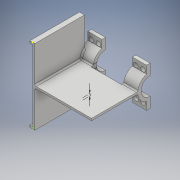
# Autodesk Inventor part: scopeHolderv2
Saved by Autodesk Inventor 2018 (Build 220112000, 112)
## iProperties
Created: 2019-03-22
Part Number: scopeHolderv2
Material: Generic
Document SubType Name: Modeling
Designer: Aditya Kendre
Density: 1 g/cm^3
Appearance: Default
Author: Aditya Kendre
## iProperties of the stored document scopeHolderv2_3DPrint.ipt
Created: 2019-03-22
Part Number: scopeHolderv2_3DPrint
Material: Generic
Document SubType Name: Modeling
Designer: Aditya Kendre
Density: 1 g/cm^3
Appearance: Default
Author: Aditya Kendre
Autodesk Inventor part; units mm, degrees
ref_plane "YZ Plane" through (0, 0, 0) normal (1, 0, 0) x (0, 1, 0)
ref_plane "XZ Plane" through (0, 0, 0) normal (0, 1, 0) x (-1, 0, 0)
ref_plane "XY Plane" through (0, 0, 0) normal (0, 0, 1) x (1, 0, 0)
sketch "Sketch1" plane through (0, 0, 0) normal (0, 1, 0) x (-1, 0, 0)
  line L0 (0, 0) -> (3, 0)
  line L1 (3, 0) -> (3, -106)
  line L2 (3, -106) -> (0, -106)
  line L3 (0, -106) -> (0, 0)
  line L4 (0, -53) -> (-80, -53) construction
  line L5 (-80, -51.5) -> (0, -51.5)
  line L6 (0, -51.5) -> (0, -54.5)
  line L7 (0, -54.5) -> (-80, -54.5)
  line L8 (-80, -54.5) -> (-80, -51.5)
  line L9 (-80, -51.5) -> (0, -54.5) construction
  line L10 (0, -51.5) -> (-80, -54.5) construction
  point P0 (-40, -53)
  dimension "d0" = 3
  dimension "d1" = 106
  dimension "d2" = 80
  dimension "d3" = 3
  constraints: 22 end point, 4 midpoint, 4 parallel, 3 horizontal, 2 perpendicular, 1 point on line
  measures "d0" distance of L1.end L2.end
  measures "d1" distance of L0.end L1.end
  measures "d2" distance of L4.start L4.end
  measures "d3" distance of L5.end L6.end
extrude "Extrusion1" add sketch "Sketch1" along normal blind 70
sketch "Sketch2" plane through (-3, 0, -106) normal (-1, 0, 0) x (0, 0, 1)
  line L0 (0, 0) -> (106, 0) projected
  line L1 (0, 70) -> (106, 70) projected
  line L2 (106, 0) -> (103, 0)
  line L3 (103, 0) -> (103, 70)
  line L4 (103, 70) -> (106, 70)
  line L5 (106, 70) -> (106, 0)
  dimension "d6" = 3
  constraints: 8 end point, 2 parallel, 1 horizontal, 1 perpendicular, 1 point on line
  measures "d6" distance of L3.end L4.end
sketch "Sketch3" plane through (-3, 0, -106) normal (-1, 0, 0) x (0, 0, 1)
  line L0 (51.5, 70) -> (0, 70) projected
  line L1 (0, 0) -> (3, 0)
  line L2 (3, 0) -> (3, 70)
  line L3 (3, 70) -> (0, 70)
  line L4 (0, 70) -> (0, 0)
  point P0 (106, 0)
  dimension "d7" = 3
  constraints: 8 end point, 2 parallel, 1 horizontal, 1 perpendicular, 1 point on line
  measures "d7" distance of L3.end L2.end
sketch "Sketch4" plane through (-3, 0, -106) normal (-1, 0, 0) x (0, 0, 1)
  line L0 (51.5, 0) -> (0, 0) projected
  line L1 (51.5, 70) -> (0, 70) projected
  line L2 (0, 0) -> (3, 0)
  line L3 (3, 0) -> (3, 70)
  line L4 (3, 70) -> (0, 70)
  line L5 (0, 70) -> (0, 0)
  point P0 (106, 0)
  dimension "d8" = 3
  constraints: 8 end point, 2 parallel, 1 horizontal, 1 perpendicular, 1 point on line
  measures "d8" distance of L4.end L3.end
extrude "Extrusion2" add sketch "Sketch2" along normal blind 4
extrude "Extrusion3" add sketch "Sketch4" along normal blind 4
sketch "Sketch5" plane through (-3, 0, -3) normal (-1, 0, 0) x (0, 0, 1)
  line L0 (-103, 0) -> (-103, 70) construction
  line L1 (-103, 70) -> (3, 70) construction
  line L2 (3, 70) -> (-50, 70) construction
  line L3 (-50, 70) -> (-50, 82.7) construction
  circle A0 centre (-50, 82.7) radius 12.7
  circle A1 centre (-50, 82.7) radius 17.5
  point P0 (3, 0)
  dimension "d13" = 12.7
  dimension "d14" = 25.4
  dimension "d15" = 35
  constraints: 6 end point, 2 centre point, 2 coincident, 1 horizontal, 1 midpoint, 1 perpendicular
  measures "d13" distance of L2.end L3.end
  measures "d14" diameter of A0
  measures "d15" diameter of A1
extrude "Extrusion4" add sketch "Sketch5" against normal blind 20
sketch "Sketch6" plane through (80, 0, -51.5) normal (1, 0, 0) x (0, 0, -1)
  circle A0 centre (1.5, 82.7) radius 12.7 projected
  circle A1 centre (1.5, 82.7) radius 12.7
  circle A2 centre (1.5, 82.7) radius 17.5
  point P0 (-51.5, 0)
  point P1 (1.5, 70)
  constraints: 2 centre point, 2 coincident, 1 vertical alignment
extrude "Extrusion5" add sketch "Sketch6" against normal blind 20
sketch "Sketch7" plane through (80, 0, -51.5) normal (1, 0, 0) x (0, 0, -1)
  arc A0 (3, 65.2644) -> (0, 65.2644) centre (1.5, 82.7) ccw projected
  line L0 (1.5, 82.7) -> (-23.0448, 82.7)
  line L1 (-23.0448, 82.7) -> (-23.0448, 99.7436)
  line L2 (-23.0448, 99.7436) -> (1.5, 99.7436)
  line L3 (1.5, 99.7436) -> (1.5, 82.7)
  line L4 (-23.0448, 82.7) -> (23.5266, 82.7)
  line L5 (23.5266, 82.7) -> (23.5266, 103.3181)
  line L6 (23.5266, 103.3181) -> (-23.0448, 103.3181)
  line L7 (-23.0448, 103.3181) -> (-23.0448, 82.7)
  point P0 (-51.5, 0)
  constraints: 16 end point, 4 parallel, 2 horizontal, 2 perpendicular
extrude "Extrusion6" cut sketch "Sketch7" against normal blind 2000
sketch "Sketch8" plane through (80, 82.7, -65.7) normal (0, 1, 0) x (1, 0, 0)
  line L0 (-83, -25.4) -> (-83, 0) projected
  line L1 (-83, 0) -> (-63, 0)
  line L2 (-63, 0) -> (-63, 15)
  line L3 (-63, 15) -> (-83, 15)
  line L4 (-83, 15) -> (-83, 0)
  line L5 (0, 0) -> (-20, 0) projected
  line L6 (0, 0) -> (-20, 0)
  line L7 (-20, 0) -> (-20, 15)
  line L8 (-20, 15) -> (0, 15)
  line L9 (0, 15) -> (0, 0)
  line L10 (-20, -25.4) -> (0, -25.4) projected
  line L11 (-20, -25.4) -> (0, -25.4)
  line L12 (0, -25.4) -> (0, -40.4)
  line L13 (0, -40.4) -> (-20, -40.4)
  line L14 (-20, -40.4) -> (-20, -25.4)
  line L15 (-83, -25.4) -> (-63, -25.4)
  line L16 (-63, -25.4) -> (-63, -40.4)
  line L17 (-63, -40.4) -> (-83, -40.4)
  line L18 (-83, -40.4) -> (-83, -25.4)
  point P0 (-80, -65.7)
  dimension "d22" = 15
  dimension "d23" = 15
  dimension "d24" = 15
  dimension "d25" = 20
  constraints: 32 end point, 8 parallel, 4 horizontal, 4 perpendicular, 4 point on line
  measures "d22" distance of L2.end L1.end
  measures "d23" distance of L6.end L7.end
  measures "d24" distance of L11.end L12.end
  measures "d25" distance of L16.end L17.end
extrude "Extrusion7" add sketch "Sketch8" against normal blind 5
fillet "Fillet1" radius 2 12 edges at (0, 32.6322, -54.5) (0, 66.7372, -60.1721) (8.5, 65.2644, -54.5) (17, 67.6322, -54.5) (70, 65.2644, -54.5) (60, 67.6322, -54.5) (0, 32.6322, -51.5) (8.5, 65.2644, -51.5) (0, 66.7372, -45.8279) (17, 67.6322, -51.5) (70, 65.2644, -51.5) (60, 67.6322, -51.5)
sketch "Sketch9" plane through (0, 70, 0) normal (0, 1, 0) x (1, 0, 0)
  arc A0 (17.0325, 56.141) -> (19, 54.5) centre (19, 56.5) ccw projected
  line L0 (60, 49.5) -> (60, 53) projected
  line L1 (17.0325, 56.141) -> (60, 56.141)
  line L2 (60, 56.141) -> (60, 49.5)
  line L3 (60, 49.5) -> (17.0325, 49.5)
  line L4 (17.0325, 49.5) -> (17.0325, 56.141)
  point P0 (0, 0)
  constraints: 8 end point, 2 parallel, 1 horizontal, 1 perpendicular
extrude "Extrusion8" cut sketch "Sketch9" against normal blind 7.5
sketch "Sketch10" plane through (-3, 82.7, -40.3) normal (0, 1, 0) x (1, 0, 0)
  line L0 (20, -4.0705) -> (20, -15) projected
  line L1 (0, 0) -> (20, 0) projected
  line L2 (20, -15) -> (0, -15)
  line L3 (0, -15) -> (0, 0)
  line L4 (0, 0) -> (20, 0)
  line L5 (20, 0) -> (20, -15)
  line L6 (20, -15) -> (0, -15) construction
  line L7 (10, -15) -> (10, 40.4) construction
  line L8 (0, 40.4) -> (20, 40.4) construction
  line L9 (0, -15) -> (10, 0) construction
  line L10 (0, 0) -> (10, -15) construction
  line L11 (20, 0) -> (10, -15) construction
  line L12 (20, -15) -> (10, 0) construction
  line L13 (20, 25.4) -> (0, 25.4) construction
  line L14 (10, 25.4) -> (0, 40.4) construction
  line L15 (0, 62.7) -> (0, -37.3) construction
  line L16 (0, 25.4) -> (10, 40.4) construction
  line L17 (10, 40.4) -> (20, 25.4) construction
  line L18 (20, 25.4) -> (15, 32.9) construction
  line L19 (20, 40.4) -> (20, 25.4) construction
  line L20 (10, 25.4) -> (20, 40.4) construction
  circle A0 centre (5, -7.5) radius 3.175
  circle A1 centre (15, -7.5) radius 3.175
  circle A2 centre (5, 32.9) radius 3.175
  circle A3 centre (15, 32.9) radius 3.175
  point P0 (3, -40.3)
  dimension "d31" = 6.35
  dimension "d32" = 6.35
  dimension "d33" = 6.35
  dimension "d34" = 6.35
  constraints: 28 end point, 8 midpoint, 8 parallel, 4 centre point, 2 point on line, 1 coincident, 1 horizontal, 1 perpendicular
  measures "d31" diameter of A0
  measures "d32" diameter of A1
  measures "d33" diameter of A2
  measures "d34" diameter of A3
extrude "Extrusion9" cut sketch "Sketch10" against normal blind 7.5 contours A0 | A1 | A2 | A3
sketch "Sketch11" plane through (60, 82.7, -40.3) normal (0, 1, 0) x (1, 0, 0)
  line L0 (20, -15) -> (0, -15) construction
  line L1 (10, -15) -> (10, 40.4) construction
  line L2 (0, 40.4) -> (20, 40.4) construction
  line L3 (0, 40.4) -> (10, 25.4) construction
  line L4 (20, 25.4) -> (0, 25.4) construction
  line L5 (5, 32.9) -> (20, 32.9) construction
  line L6 (20, 40.4) -> (20, 29.4705) construction
  line L7 (10, 25.4) -> (20, 40.4) construction
  line L8 (0, -15) -> (10, 0) construction
  line L9 (0, 0) -> (20, 0) construction
  line L10 (0, 0) -> (10, -15) construction
  line L11 (20, 0) -> (20, -15) construction
  line L12 (10, -15) -> (20, 0) construction
  line L13 (20, 0) -> (10, 0) construction
  line L14 (20, -15) -> (10, 0) construction
  circle A0 centre (5, -7.5) radius 3.175
  circle A1 centre (15, -7.5) radius 3.175
  circle A2 centre (5, 32.9) radius 3.175
  circle A3 centre (15, 32.9) radius 3.175
  point P0 (-60, -40.3)
  dimension "d37" = 6.35
  dimension "d38" = 6.35
  dimension "d39" = 6.35
  dimension "d40" = 6.35
  constraints: 18 end point, 7 midpoint, 4 centre point, 2 parallel, 1 coincident, 1 horizontal, 1 perpendicular, 1 point on line
  measures "d37" diameter of A0
  measures "d38" diameter of A1
  measures "d39" diameter of A2
  measures "d40" diameter of A3
extrude "Extrusion10" cut sketch "Sketch11" against normal blind 7.5
body "Solid1"
